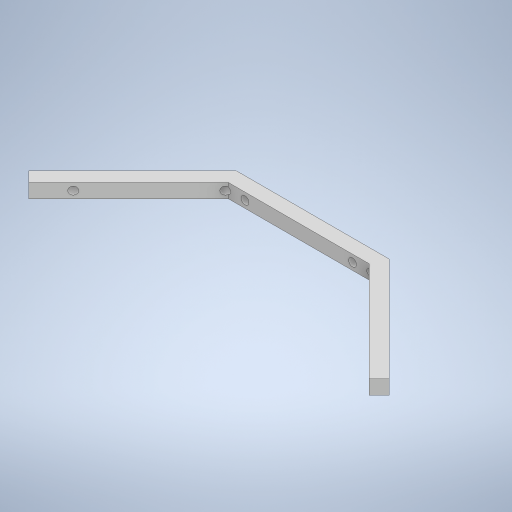
# Autodesk Inventor part: Držák TF-Luna
Saved by Autodesk Inventor 2024 (Build 280153000, 153)
## iProperties
Created: 2023-11-01
Part Number: Držák TF-Luna
Material: Všeobecné
Document SubType Name: Modeling
Designer: 42060
Density: 1 g/cm^3
Appearance: Výchozí
Author: 42060
Autodesk Inventor part; units mm, degrees
ref_plane "YZ Plane" through (0, 0, 0) normal (1, 0, 0) x (0, 1, 0)
ref_plane "XZ Plane" through (0, 0, 0) normal (0, 1, 0) x (-1, 0, 0)
ref_plane "XY Plane" through (0, 0, 0) normal (0, 0, 1) x (1, 0, 0)
sketch "Náčrt1" plane through (0, 0, 0) normal (0, 0, 1) x (1, 0, 0)
  line L0 (0, 0) -> (21.6569, 0)
  line L1 (21.6569, 0) -> (51.1127, -29.4558)
  line L2 (51.1127, -29.4558) -> (48.2843, -32.2843)
  line L3 (48.2843, -32.2843) -> (20, -4)
  line L4 (20, -4) -> (0, -4)
  line L5 (0, -4) -> (0, 0)
  dimension "d0" = 4
  dimension "d1" = 135
  dimension "d2" = 40
  dimension "d3" = 20
  constraints: 12 end point, 3 perpendicular, 1 equal length, 1 horizontal, 1 parallel
  measures "d0" distance of L4.end L0.start
  measures "d1" angle of L3 L4
  measures "d2" distance of L2.end L3.end
  measures "d3" distance of L3.end L4.end
extrude "Vysunutí1" add sketch "Náčrt1" along normal blind 4
sketch "Náčrt2" plane through (0, -4, 0) normal (0, -1, 0) x (1, 0, 0)
  line L0 (0, 0) -> (0, 4) projected
  point P0 (15.25, 2)
  point P1 (0, 2)
  dimension "d6" = 15.25
  constraints: 1 horizontal alignment, 1 midpoint
  measures "d6" distance from line of L0 point (15.25, 2)
hole "Díra1" at (15.25, -4, 2) direction (0, 1, 0) diameter 2.2 end through all
sketch "Náčrt3" plane through (48.2843, -32.2843, 4) normal (-0.7071068, -0.7071068, 0) x (-0.7071068, 0.7071068, 0)
  line L0 (0, 4) -> (0, 0) projected
  line L1 (41.6569, 4) -> (41.6569, 0) projected
  point P0 (56.9706, 4)
  point P1 (39.4069, 2)
  point P2 (8.9069, 2)
  point P3 (0, 2)
  dimension "d14" = 30.5
  dimension "d23" = 2.25
  constraints: 2 horizontal alignment, 1 midpoint
  measures "d14" distance of point (8.907, 2) point (39.407, 2)
  measures "d23" distance from line of point (39.407, 2) L1
hole "Díra2" at (20.4194, -4.4194, 2) at (41.9862, -25.9862, 2) direction (-0.7071068, -0.7071068, 0) diameter 2.2 end through all both
mirror "Zrcadlit1" about plane through (0, 0, 0) normal (1, 0, 0)
